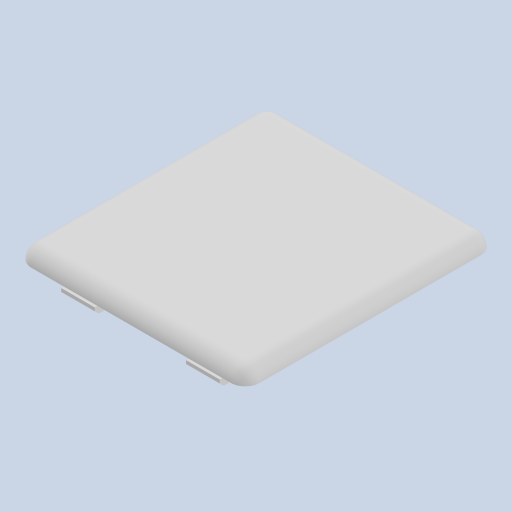
# Autodesk Inventor part: capac baterie
Saved by Autodesk Inventor 2024 (Build 280153000, 153)
## iProperties
Created: 2024-04-23
Part Number: capac baterie
Material: Generic
Document SubType Name: Modeling
Designer: mirun
Density: 1 g/cm^3
Appearance: Default
Author: mirun
Autodesk Inventor part; units mm, degrees
ref_plane "YZ Plane" through (0, 0, 0) normal (1, 0, 0) x (0, 1, 0)
ref_plane "XZ Plane" through (0, 0, 0) normal (0, 1, 0) x (-1, 0, 0)
ref_plane "XY Plane" through (0, 0, 0) normal (0, 0, 1) x (1, 0, 0)
sketch "Sketch1" plane through (0, 0, 0) normal (0, 1, 0) x (-1, 0, 0)
  line L0 (23.75, 26) -> (-23.75, 26)
  line L1 (-23.75, 26) -> (-23.75, -26)
  line L2 (-23.75, -26) -> (23.75, -26)
  line L3 (23.75, -26) -> (23.75, 26)
  line L4 (23.75, 26) -> (-23.75, -26) construction
  line L5 (-23.75, 26) -> (23.75, -26) construction
  point P0 (0, 0)
  point P1 (0, -26)
  dimension "d0" = 47.5
  dimension "d1" = 52
  constraints: 12 end point, 3 midpoint, 2 parallel, 1 horizontal, 1 perpendicular
  measures "d0" distance between parallel lines of L1 L3
  measures "d1" distance from line of L0 point (0, -26)
extrude "Extrusion1" add sketch "Sketch1" along normal blind 3
fillet "Fillet1" radius 3 4 edges at (0, 3, -26) (-23.75, 3, 0) (0, 3, 26) (23.75, 3, 0)
sketch "Sketch2" plane through (0, 0, 0) normal (0, -1, 0) x (1, 0, 0)
  line L0 (-23.75, -26) -> (-23.75, 26) construction
  line L1 (23.75, -26) -> (-23.75, -26) construction
  line L2 (21, 23.25) -> (-21, 23.25)
  line L3 (-21, 23.25) -> (-21, -23.25)
  line L4 (-21, -23.25) -> (21, -23.25)
  line L5 (21, -23.25) -> (21, 23.25)
  line L6 (21, 23.25) -> (-21, -23.25) construction
  line L7 (-21, 23.25) -> (21, -23.25) construction
  line L8 (16.5, -23.25) -> (9.5, -23.25)
  line L9 (9.5, -23.25) -> (9.5, -21.75)
  line L10 (9.5, -21.75) -> (16.5, -21.75)
  line L11 (16.5, -21.75) -> (16.5, -23.25)
  point P0 (0, 0)
  dimension "d5" = 2.75
  dimension "d6" = 2.75
  dimension "d7" = 7
  dimension "d8" = 1.5
  dimension "d9" = 9.5
  constraints: 20 end point, 4 parallel, 2 horizontal, 2 midpoint, 2 perpendicular, 1 point on line
  measures "d5" distance between parallel lines of L4 L1
  measures "d6" distance between parallel lines of L0 L3
  measures "d7" distance of L9.end L10.end
  measures "d8" distance of L8.end L9.end
  measures "d9" distance from line of L9 point (0, 0)
extrude "Extrusion2" add sketch "Sketch2" along normal blind 4 contours L4 L9 L10 L11
sketch "Sketch3" plane through (16.5, 0, -23.25) normal (0, 0, -1) x (-1, 0, 0)
  line L0 (7, 0) -> (7, -4) construction
  line L1 (0, -4) -> (7, -4)
  line L2 (7, -4) -> (7, -2.5)
  line L3 (7, -2.5) -> (0, -2.5)
  line L4 (0, -2.5) -> (0, -4)
  point P0 (16.5, 0)
  dimension "d12" = 1.5
  constraints: 8 end point, 2 parallel, 1 horizontal, 1 perpendicular, 1 point on line
  measures "d12" distance of L2.end L1.end
extrude "Extrusion3" add sketch "Sketch3" along normal blind 0.8
chamfer "Chamfer1" distance 0.8 angle 45 1 edges at (13, -4, -24.05)
fillet "Fillet2" radius 3 4 edges at (22.8713, 2.1213, 25.1213) (-22.8713, 2.1213, 25.1213) (-22.8713, 2.1213, -25.1213) (22.8713, 2.1213, -25.1213)
mirror "Mirror1" about plane through (0, 0, 0) normal (1, 0, 0) of "Extrusion2", "Chamfer1", "Extrusion3"
mirror "Mirror2" about plane through (0, 0, 0) normal (0, 0, 1) of "Extrusion2", "Chamfer1", "Extrusion3", "Mirror1"
body "Solid1"
